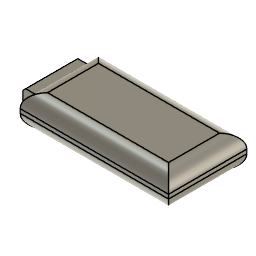
BATERIA v2 (Autodesk Fusion 360 design; units mm, degrees)
Autodesk Fusion 360 part; units mm, degrees
sketch "Boceto1" plane through (0, 0, 0) normal (0, 0, 1) x (1, 0, 0)
  line L0 (0, 0) -> (54, 0)
  line L1 (54, 0) -> (54, 28.5)
  line L2 (54, 28.5) -> (0, 28.5)
  line L3 (0, 28.5) -> (0, 0)
  dimension "d1" = 54
  dimension "d2" = 28.5
  constraint horizontal L0
  constraint vertical L1
  constraint horizontal L2
  constraint vertical L3
  constraint coincident L0.start L3.end
  measures "d1" distance of L0.start L0.end
  measures "d2" distance of L0.start L2.end
extrude "Extruir1" add sketch "Boceto1" along normal blind 11.5
fillet "Empalme1" radius 5 2 faces at (18, 9.5, 11.5) (18, 9.5, 0)
sketch "Boceto2" plane through (0, 0, 0) normal (-1, 0, 0) x (0, -1, 0)
  line L0 (-28.5, 5) -> (0, 5)
  line L1 (0, 5) -> (0, 6.5)
  line L2 (0, 6.5) -> (-28.5, 6.5)
  line L3 (-28.5, 6.5) -> (-28.5, 5)
  line L4 (-25, 2.75) -> (-5, 2.75)
  line L5 (-5, 2.75) -> (-5, 8.75)
  line L6 (-5, 8.75) -> (-25, 8.75)
  line L7 (-25, 8.75) -> (-25, 2.75)
  dimension "d7" = 5
  dimension "d8" = 20
  dimension "d9" = 6
  dimension "d10" = 2.75
  constraint horizontal L4
  constraint vertical L5
  constraint horizontal L6
  constraint vertical L7
  measures "d7" distance of L1 L5
  measures "d8" distance of L4.start L4.end
  measures "d9" distance of L4.end L5.end
  measures "d10" distance of origin L4
extrude "Extruir2" add sketch "Boceto2" along normal blind 4 and the other way blind 1 contours L0 L2 L5 L7 | L0 L4 L5 L7 | L2 L5 L6 L7
chamfer "Chaflán1" distance 1 angle 45 5 edges at (-1.7326, 25, 8.75) (-1.7326, 25, 2.75) (-4, 15, 8.75) (-4, 15, 2.75) (-4, 25, 5.75)
equation "d10 = ( ( 11.5 - 6 ) / 2 ) * 1 mm"
